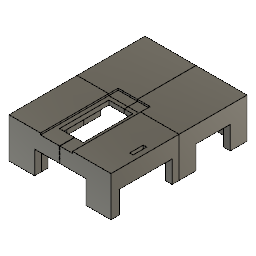
stands for wormbot (v15~recovered) (Autodesk Fusion 360 design; units mm, degrees)
Autodesk Fusion 360 part; units mm, degrees
note: some values were not read from the file. Set by a fixed rule: which face or edge a step refers to.
box "BoxPrimitive1" add length 381 width 305 height 5 placed x (0, 1, 0) y (-1, 0, 0) z (0, 0, 1) at (0, 0, 0) makes body 1
extrude "Extrude1" add 1 faces at (-203.3333, 127, 5) along direction (0, 0, 1) blind 113 on bodies 1 bodies 1
extrude "Extrude2" cut 1 faces at (0, 254, 39.3333) along direction (-1, 0, 0) blind 152.5 on bodies 1 bodies 1
extrude "Extrude3" cut 1 faces at (-203.3333, 0, 39.3333) along direction (0, 1, 0) blind 190.5 on bodies 1 bodies 1
shell "Shell1" thickness 20 removed faces 1 at (-254.1667, 254, 118) on bodies 1
extrude "Extrude4" add 1 faces at (-247.5, 260.6667, 20) along direction (0, 0, 1) blind 20 on bodies 1 bodies 1
sketch "Sketch2" plane through (0, 0, 0) normal (0, 0, 1) x (1, 0, 0)
  line L0 (0, 0) -> (150, 0)
  line L1 (150, 0) -> (150, 200)
  line L2 (150, 200) -> (0, 200)
  line L3 (0, 200) -> (0, 0)
  dimension "d15" = 150
  dimension "d16" = 200
  constraint horizontal L0
  constraint vertical L1
  constraint horizontal L2
  constraint vertical L3
  constraint coincident L0.start L3.end
  measures "d15" distance of L0.start L0.end
  measures "d16" distance of L0 L2
move_body "Move1" bodies 1 to x (1, 0, 0) y (0, 1, 0) z (0, 0, 1) at (110, -190, 0)
extrude "Extrude5" add sketch "Sketch2" along normal blind 118 separate body makes body 2
shell "Shell2" thickness 20 removed faces 1 at (50, 133.3333, 118) on bodies 2
copy_body "CopyPasteBodies1" bodies 2 makes body 3
move_body "Move2" bodies 3 to x (1, 0, 0) y (0, 1, 0) z (0, 0, 1) at (175, 0, 0)
copy_body "CopyPasteBodies2" bodies 3 2 makes body 4 makes body 5
move_body "Move3" bodies 4 5 to x (1, 0, 0) y (0, 1, 0) z (0, 0, 1) at (0, 225, 0)
sketch "Sketch4" plane through (0, 0, 118) normal (0, 0, 1) x (-1, 0, 0)
  line L0 (-20, -405) -> (-130, -405)
  line L1 (-130, -405) -> (-130, -245)
  line L2 (-130, -245) -> (-20, -245)
  line L3 (-20, -245) -> (-20, -405)
  line L4 (0, -425) -> (0, -225)
  line L5 (0, -225) -> (-150, -225)
  line L6 (-150, -225) -> (-150, -425)
  line L7 (-150, -425) -> (0, -425)
  line L8 (-150, -225) -> (-20, -225)
  line L9 (-20, -225) -> (-20, -405)
  line L10 (-20, -405) -> (-150, -405)
  line L11 (-150, -405) -> (-150, -225)
  constraint horizontal L8
  constraint vertical L9
  constraint horizontal L10
  constraint vertical L11
  constraint coincident L0.start L3.end
  constraint coincident L5.end L6.start
sketch "Sketch5" plane through (0, 0, 118) normal (0, 0, 1) x (-1, 0, 0)
  line L0 (-195, -405) -> (-305, -405)
  line L1 (-305, -405) -> (-305, -245)
  line L2 (-305, -245) -> (-195, -245)
  line L3 (-195, -245) -> (-195, -405)
  line L4 (-175, -425) -> (-175, -225)
  line L5 (-175, -225) -> (-325, -225)
  line L6 (-325, -225) -> (-325, -425)
  line L7 (-325, -425) -> (-175, -425)
  line L8 (-175, -225) -> (-305, -225)
  line L9 (-305, -225) -> (-305, -405)
  line L10 (-305, -405) -> (-175, -405)
  line L11 (-175, -405) -> (-175, -225)
  constraint horizontal L8
  constraint vertical L9
  constraint horizontal L10
  constraint vertical L11
  constraint coincident L0.end L1.start
  constraint coincident L4.end L5.start
sketch "Sketch6" plane through (0, 0, 118) normal (0, 0, 1) x (-1, 0, 0)
  line L0 (-20, -180) -> (-130, -180)
  line L1 (-130, -180) -> (-130, -20)
  line L2 (-130, -20) -> (-20, -20)
  line L3 (-20, -20) -> (-20, -180)
  line L4 (0, -200) -> (0, 0)
  line L5 (0, 0) -> (-150, 0)
  line L6 (-150, 0) -> (-150, -200)
  line L7 (-150, -200) -> (0, -200)
  line L8 (-150, -200) -> (-20, -200)
  line L9 (-20, -200) -> (-20, -20)
  line L10 (-20, -20) -> (-150, -20)
  line L11 (-150, -20) -> (-150, -200)
  constraint horizontal L8
  constraint vertical L9
  constraint horizontal L10
  constraint vertical L11
  constraint coincident L2.end L3.start
  constraint coincident L6.end L7.start
sketch "Sketch7" plane through (0, 0, 118) normal (0, 0, 1) x (-1, 0, 0)
  line L0 (-195, -180) -> (-305, -180)
  line L1 (-305, -180) -> (-305, -20)
  line L2 (-305, -20) -> (-195, -20)
  line L3 (-195, -20) -> (-195, -180)
  line L4 (-175, -200) -> (-175, 0)
  line L5 (-175, 0) -> (-325, 0)
  line L6 (-325, 0) -> (-325, -200)
  line L7 (-325, -200) -> (-175, -200)
  line L8 (-175, -200) -> (-305, -200)
  line L9 (-305, -200) -> (-305, -20)
  line L10 (-305, -20) -> (-175, -20)
  line L11 (-175, -20) -> (-175, -200)
  constraint horizontal L8
  constraint vertical L9
  constraint horizontal L10
  constraint vertical L11
  constraint coincident L1.end L2.start
  constraint coincident L4.start L7.end
extrude "Extrude6" cut sketch "Sketch5" sketch "Sketch6" sketch "Sketch4" sketch "Sketch7" against normal blind 100 contours L2 L3 L4 L5 L8 L9 L10 L11 of sketch 2 contours L0 L1 L6 L7 L8 L9 L10 L11 of sketch 3 contours L1 L2 L5 L6 L8 L9 L10 L11 of sketch 4 contours L0 L3 L4 L7 L8 L9 L10 L11 bodies 2 3 4 5
move_body "Move4" bodies 3 2 to x (1, 0, 0) y (0, 1, 0) z (0, 0, 1) at (0, 25, 0)
move_body "Move5" bodies 4 3 to x (1, 0, 0) y (0, 1, 0) z (0, 0, 1) at (-25, 0, 0)
move_body "Move6" bodies 2 4 5 3 to x (1, 0, 0) y (0, -1, 0) z (0, 0, -1) at (-150, 225, 36)
other "Base Mesh Feature1"
move_body "Move7" bodies 5 2 4 3 to x (1, 0, 0) y (0, 1, 0) z (0, 0, 1) at (0, 1.0624, 83.0011)
other "Modify1"
ref_plane "WorkPlane1" through (0, 225, 0) normal (0, 1, 0) x (0, 0, 1)
ref_plane "WorkPlane2" through (0, -600, 0) normal (0, 1, 0) x (0, 0, 1)
ref_plane "WorkPlane3" through (-325, 0, 0) normal (1, 0, 0) x (0, 1, 0)
ref_plane "WorkPlane4" through (0, 0, 650) normal (0, 0, 1) x (1, 0, 0)
ref_plane "WorkPlane5" through (0, 0, -100) normal (0, 0, 1) x (1, 0, 0)
move_body "Move8" bodies 4 3 to x (1, 0, 0) y (0, 1, 0) z (0, 0, 1) at (50, 0, 0)
move_body "Move9" bodies 2 3 to x (1, 0, 0) y (0, 1, 0) z (0, 0, 1) at (0, 70, 0)
extrude "Extrude9" cut 4 faces at (106.6667, 197.7291, 99.0011) (-93.3333, 197.7291, 99.0011) (-93.3333, -125.6042, 99.0011) (106.6667, -125.6042, 99.0011) along direction (0, 0, 1) blind 2 on bodies 2 3 4 5 bodies 2 3 4 5
sketch "Sketch9" plane through (0, -178.9376, 0) normal (0, 1, 0) x (-1, 0, 0)
  line L0 (-180, 101.0011) -> (-180, 1.0011)
  line L1 (-180, 1.0011) -> (-50, 1.0011)
  line L2 (-50, 1.0011) -> (-50, 101.0011)
  line L3 (-50, 101.0011) -> (-180, 101.0011)
  line L4 (-180, 60) -> (-124.686, 101.0011)
  line L5 (-180, 101.0011) -> (-124.686, 101.0011)
  line L6 (-180, 101.0011) -> (-180, 60)
  constraint coincident L0 L4.start
  constraint coincident L3 L4.end
  constraint coincident L0.start L3.end
move_body "Move10" bodies 2 3 to x (1, 0, 0) y (0, 1, 0) z (0, 0, 1) at (0, -70, 0)
move_body "Move11" bodies 3 4 to x (1, 0, 0) y (0, 1, 0) z (0, 0, 1) at (-50, 0, 0)
other "Base Mesh Feature2"
other "Modify2"
sketch "Sketch10" plane through (0, 0, 119.0011) normal (0, 0, 1) x (-1, 0, 0)
  line L0 (150, -1.0624) -> (150, 198.9376)
  line L1 (150, 198.9376) -> (0, 198.9376)
  line L2 (0, 198.9376) -> (0, -1.0624)
  line L3 (0, -1.0624) -> (150, -1.0624)
  line L4 (56.575, -28.8666) -> (-35, -28.8666)
  line L5 (-35, -28.8666) -> (-35, 205)
  line L6 (-35, 205) -> (56.575, 205)
  line L7 (56.575, 205) -> (56.575, -28.8666)
  line L8 (45, 10) -> (-25, 10)
  line L9 (-25, 10) -> (-25, 155)
  line L10 (-25, 155) -> (45, 155)
  line L11 (45, 155) -> (45, 10)
  constraint horizontal L4
  constraint vertical L5
  constraint horizontal L6
  constraint vertical L7
  constraint horizontal L8
  constraint vertical L9
  constraint horizontal L10
  constraint vertical L11
extrude "Extrude10" cut sketch "Sketch10" against normal blind 5 contours L1 L2 L3 L4 L5 L6 L7 L8 L9 L10 | L1 L2 L3 L7 L8 L10 L11 bodies 2 3 4 5
extrude "Extrude11" cut 2 faces at (-30, -106.6667, 119.0011) (8.3333, -106.6667, 119.0011) along direction (0, 0, -1) blind 10 on bodies 4 5 bodies 4 5
extrude "Extrude12" cut 1 faces at (-30, -106.6667, 109.0011) along direction (0, 0, -1) blind 30 on bodies 5 bodies 5
extrude "Extrude13" cut 1 faces at (8.3333, -106.6667, 109.0011) along direction (0, 0, -1) blind 100 on bodies 4 bodies 4
extrude "Extrude14" cut 2 faces at (35, 10.3305, 115.6678) (35, -65.6042, 117.3345) along direction (1, 0, 0) blind 2 on bodies 3 4 bodies 3 4
move_body "Move12" bodies 2 3 4 5 to x (1, 0, 0) y (0, 1, 0) z (0, 0, 1) at (0, 50, 0)
other "Modify3"
sketch "Sketch12" plane through (150, 0, 0) normal (1, 0, 0) x (0, 1, 0)
  line L0 (51.0624, 119.0011) -> (-148.9376, 119.0011)
  line L1 (-148.9376, 119.0011) -> (-148.9376, 1.0011)
  line L2 (-148.9376, 1.0011) -> (51.0624, 1.0011)
  line L3 (51.0624, 1.0011) -> (51.0624, 119.0011)
  line L4 (-129.1971, 16.38) -> (50.8029, 16.38)
  line L5 (50.8029, 16.38) -> (50.8029, 1.38)
  line L6 (50.8029, 1.38) -> (-129.1971, 1.38)
  line L7 (-129.1971, 1.38) -> (-129.1971, 16.38)
  dimension "d65" = 180
  dimension "d66" = 15
  constraint horizontal L4
  constraint vertical L5
  constraint horizontal L6
  constraint vertical L7
  measures "d65" distance of L4.start L4.end
  measures "d66" distance of L4.start L6.end
extrude "Extrude18" cut sketch "Sketch12" against normal blind 30 contours L4 L5 L6 L7 bodies 4
extrude "Extrude19" cut 1 faces at (143.3333, -69.1106, 1.38) along direction (0, 0, -1) blind 10 on bodies 4 bodies 4
sketch "Sketch13" plane through (130, 0, 0) normal (-1, 0, 0) x (0, -1, 0)
  line L0 (-50.8029, 1.0011) -> (-50.8029, 16.38)
  line L1 (-50.8029, 16.38) -> (128.9376, 16.38)
  line L2 (128.9376, 16.38) -> (128.9376, 101.0011)
  line L3 (128.9376, 101.0011) -> (-51.0624, 101.0011)
  line L4 (-51.0624, 101.0011) -> (-51.0624, 1.0011)
  line L5 (-51.0624, 1.0011) -> (-50.8029, 1.0011)
  line L6 (-50.6729, 64.0011) -> (128.9376, 64.0011)
  line L7 (128.9376, 64.0011) -> (128.9376, 59.0011)
  line L8 (128.9376, 59.0011) -> (-50.6729, 59.0011)
  line L9 (-50.6729, 59.0011) -> (-50.6729, 64.0011)
  point P0 (-50.6729, 64.0011)
  dimension "d71" = 5
  constraint horizontal L6
  constraint vertical L7
  constraint horizontal L8
  constraint vertical L9
  constraint coincident P0 L6.start
  measures "d71" distance of P0 L8.end
extrude "Extrude22" cut 1 faces at (143.3333, -69.1106, 16.38) along direction (0, 0, 1) blind 50 on bodies 4 bodies 4
sketch "Pegs 1" plane through (0, 51.0624, 0) normal (0, 1, 0) x (-1, 0, 0)
  line L0 (-37, 114.0011) -> (-37, 119.0011)
  line L1 (-37, 119.0011) -> (-150, 119.0011)
  line L2 (-150, 119.0011) -> (-150, 1.0011)
  line L3 (-150, 1.0011) -> (-130, 1.0011)
  line L4 (-130, 1.0011) -> (-130, 101.0011)
  line L5 (-130, 101.0011) -> (0, 101.0011)
  line L6 (0, 101.0011) -> (0, 114.0011)
  line L7 (0, 114.0011) -> (-37, 114.0011)
  circle A0 centre (-110, 110) radius 5
  circle A1 centre (-140, 79.0011) radius 5
  circle A2 centre (-140, 39.0011) radius 5
  line L8 (0, 20) -> (0, 2.5)
  circle A3 centre (110, 110) radius 5
  circle A4 centre (140, 79.0011) radius 5
  circle A5 centre (140, 39.0011) radius 5
  circle A6 centre (110, 110) radius 4.75
  circle A7 centre (140, 79.0011) radius 4.75
  circle A8 centre (-140, 39.0011) radius 4.75
  circle A9 centre (-110, 110) radius 4.75
  circle A10 centre (-140, 79.0011) radius 4.75
  circle A11 centre (140, 39.0011) radius 4.75
  dimension "d78" = 40
  dimension "d79" = 10
  dimension "d80" = 40
  dimension "d81" = 10
  dimension "d82" = 40
  dimension "d111" = 9.5
  dimension "d112" = 9.5
  dimension "d113" = 9.5
  dimension "d114" = 9.5
  dimension "d115" = 9.5
  dimension "d116" = 9.5
  constraint symmetric A0 L8 A3
  constraint symmetric A1 L8 A4
  constraint symmetric A2 L8 A5
  constraint concentric A3 A6
  constraint concentric A4 A7
  constraint concentric A2 A8
  constraint concentric A0 A9
  constraint concentric A1 A10
  constraint concentric A5 A11
  measures "d78" distance of L2 A0.centre
  measures "d79" diameter of A1
  measures "d80" distance of L1 A1.centre
  measures "d81" diameter of A2
  measures "d82" distance of A1.centre A2.centre
  measures "d111" diameter of A6
  measures "d112" diameter of A7
  measures "d113" diameter of A8
  measures "d114" diameter of A9
  measures "d115" diameter of A10
  measures "d116" diameter of A11
extrude "Extrude23" cut sketch "Pegs 1" along normal blind 10 contours A0 | A1 | A2 | A3 | A4 | A5 | A6 | A7 | A8 | A9 | A10 | A11 bodies 2 3
move_body "Move13" bodies 2 3 to x (1, 0, 0) y (0, 1, 0) z (0, 0, 1) at (0, 50, 0)
extrude "Extrude24" add sketch "Pegs 1" along normal blind 9 contours A6 | A7 | A8 | A9 | A10 | A11 bodies 4 5
move_body "Move14" bodies 2 3 to x (1, 0, 0) y (0, 1, 0) z (0, 0, 1) at (0, -50, 0)
move_body "Move15" bodies 4 3 to x (1, 0, 0) y (0, 1, 0) z (0, 0, 1) at (50, -50.6352, 0.073)
move_body "Move16" bodies 4 5 to x (1, 0, 0) y (0, 1, 0) z (0, 0, 1) at (0, -50, 0)
move_body "Move17" bodies 4 to x (1, 0, 0) y (0, 1, 0) z (0, 0, 1) at (0, 50, 0)
move_body "Move18" bodies 2 to x (1, 0, 0) y (0, 1, 0) z (0, 0, 1) at (0, -50, 0)
sketch "Sketch17" plane through (50, 0, 0) normal (-1, 0, 0) x (0, -1, 0)
  line L0 (-0.4273, 114.0741) -> (-28.2314, 114.0741)
  line L1 (-28.2314, 114.0741) -> (-28.2314, 119.0741)
  line L2 (-28.2314, 119.0741) -> (-200.4273, 119.0741)
  line L3 (-200.4273, 119.0741) -> (-200.4273, 1.0741)
  line L4 (-200.4273, 1.0741) -> (-180.4273, 1.0741)
  line L5 (-180.4273, 1.0741) -> (-180.4273, 101.0741)
  line L6 (-180.4273, 101.0741) -> (-0.4273, 101.0741)
  line L7 (-0.4273, 101.0741) -> (-0.4273, 114.0741)
  circle A0 centre (169.5727, 107.9826) radius 5
  line L8 (199.5727, 114.0741) -> (199.5727, 1.0741)
  circle A1 centre (190, 74.0741) radius 5
  line L9 (199.5727, 114.0741) -> (155.6352, 114.0741)
  circle A2 centre (190.1387, 34.0741) radius 5
  line L10 (0, 2.5) -> (0, 20)
  circle A3 centre (-190.1387, 34.0741) radius 5
  circle A4 centre (-190, 74.0741) radius 5
  circle A5 centre (-169.5727, 107.9826) radius 5
  circle A6 centre (169.5727, 107.9826) radius 3.5
  circle A7 centre (190, 74.0741) radius 3.5
  circle A8 centre (190.1387, 34.0741) radius 3.5
  circle A9 centre (-169.5727, 107.9826) radius 3.5
  circle A10 centre (-190, 74.0741) radius 3.5
  circle A11 centre (-190.1387, 34.0741) radius 3.5
  dimension "d93" = 10
  dimension "d94" = 30
  dimension "d95" = 10
  dimension "d96" = 40
  dimension "d97" = 10
  dimension "d98" = 40
  dimension "d117" = 7
  dimension "d118" = 7
  dimension "d119" = 7
  dimension "d120" = 7
  dimension "d121" = 7
  dimension "d122" = 7
  constraint symmetric A0 L10 A5
  constraint symmetric A1 L10 A4
  constraint symmetric A2 L10 A3
  constraint concentric A0 A6
  constraint concentric A1 A7
  constraint concentric A2 A8
  constraint concentric A5 A9
  constraint concentric A4 A10
  constraint concentric A3 A11
  measures "d93" diameter of A0
  measures "d94" distance of A0.centre L8
  measures "d95" diameter of A1
  measures "d96" distance of A1.centre L9
  measures "d97" diameter of A2
  measures "d98" vertical distance of A1.centre A2.centre
  measures "d117" diameter of A6
  measures "d118" diameter of A7
  measures "d119" diameter of A8
  measures "d120" diameter of A9
  measures "d121" diameter of A10
  measures "d122" diameter of A11
move_body "Move19" bodies 2 5 to x (1, 0, 0) y (0, 1, 0) z (0, 0, 1) at (50, 0, 0)
move_body "Move20" bodies 4 3 to x (1, 0, 0) y (0, 1, 0) z (0, 0, 1) at (0, 0.639, 0)
extrude "Extrude25" cut sketch "Sketch17" along normal blind 10 contours A0 | A1 | A2 | A3 | A4 | A5 | A6 | A7 | A8 | A9 | A10 | A11 bodies 2 5
extrude "Extrude26" add sketch "Sketch17" along normal blind 10 contours A6 | A7 | A8 | A9 | A10 | A11 bodies 3 4
move_body "Move21" bodies 2 4 5 3 to x (1, 0, 0) y (0, -1, 0) z (0, 0, -1) at (0, 2.1325, 128.1482)
move_body "Move22" bodies 3 2 to x (1, 0, 0) y (0, 1, 0) z (0, 0, 1) at (0, -25, 0)
move_body "Move23" bodies 3 4 to x (1, 0, 0) y (0, 1, 0) z (0, 0, 1) at (25, 0, 0)
extrude "Extrude27" add 1 faces at (218.3333, 1.3258, 83.4882) along direction (0, 1, 0) blind 30 on bodies 4 bodies 4
move_body "Move24" bodies 5 3 2 4 to x (1, 0, 0) y (0, -1, 0) z (0, 0, -1) at (0, 2.1402, 124.2941)
move_body "Move25" bodies 2 3 4 5 to x (1, 0, 0) y (0, 1, 0) z (0, 0, 1) at (-49.8589, 23.9323, 0)
move_body "Move26" bodies 2 3 to x (1, 0, 0) y (0, 1, 0) z (0, 0, 1) at (0, -25, 0)
move_body "Move27" bodies 4 3 to x (1, 0, 0) y (0, 1, 0) z (0, 0, 1) at (-25, 0, 0)
move_body "Move28" bodies 2 5 3 4 to x (1, 0, 0) y (0, 1, 0) z (0, 0, 1) at (-1.1259, 26.5865, 0)
sketch "Sketch18" plane through (0, 0, 0) normal (0, 0, 1) x (1, 0, 0)
  line L0 (-266.1691, -475) -> (159.4864, -475)
  line L1 (159.4864, -475) -> (159.4864, 284.4296)
  line L2 (159.4864, 284.4296) -> (-266.1691, 284.4296)
  line L3 (-266.1691, 284.4296) -> (-266.1691, -475)
  constraint horizontal L0
  constraint vertical L1
  constraint horizontal L2
  constraint vertical L3
other "Base Mesh Feature4"
other "Modify4"
other "Base Mesh Feature5"
other "Modify5"
extrude "Extrude28" add sketch "Sketch18" against normal blind 30 separate body makes body 6
extrude "Extrude29" add 1 faces at (159.4864, -221.8568, -10) along direction (1, 0, 0) blind 50 on bodies 6 bodies 6
sketch "Sketch19" plane through (0, 0, 0) normal (0, 0, 1) x (1, 0, 0)
  line L0 (-258.0781, -43.3) -> (-233.0723, -43.3)
  line L1 (-233.0723, -43.3) -> (-233.0723, -17.8396)
  line L2 (-233.0723, -17.8396) -> (-258.0781, -17.8396)
  line L3 (-258.0781, -17.8396) -> (-258.0781, -43.3)
  constraint horizontal L0
  constraint vertical L1
  constraint horizontal L2
  constraint vertical L3
extrude "Extrude30" add sketch "Sketch19" along normal blind 15 separate body makes body 7
move_body "Move29" bodies 3 4 to x (1, 0, 0) y (0, 1, 0) z (0, 0, 1) at (30, 0, 0)
move_body "Move30" bodies 2 3 to x (1, 0, 0) y (0, 1, 0) z (0, 0, 1) at (0, 40, 0)
move_body "Move31" bodies 2 3 4 5 to x (1, 0, 0) y (0, -1, 0) z (0, 0, -1) at (0, 183.1777, -5.7059)
move_body "Move32" bodies 4 5 to x (1, 0, 0) y (0, 1, 0) z (0, 0, 1) at (0, -40, 0)
move_body "Move33" bodies 4 3 to x (1, 0, 0) y (0, 1, 0) z (0, 0, 1) at (-30, 0, 0)
move_body "Move34" bodies 2 4 5 3 to x (1, 0, 0) y (0, -1, 0) z (0, 0, -1) at (0, 143.1777, -5.7059)
sketch "Sketch20" plane through (0, -148.4112, 0) normal (0, -1, 0) x (1, 0, 0)
  line L0 (-0.9847, 110.1471) -> (-57.5597, 110.1471)
  line L1 (-57.5597, 110.1471) -> (-57.5597, 115.1471)
  line L2 (-57.5597, 115.1471) -> (-150.9847, 115.1471)
  line L3 (-150.9847, 115.1471) -> (-150.9847, -2.8529)
  line L4 (-150.9847, -2.8529) -> (-0.9847, -2.8529)
  line L5 (-0.9847, -2.8529) -> (-0.9847, 110.1471)
  line L6 (0, 0) -> (-75, 0)
  line L7 (-75, 0) -> (-75, 65.379)
  line L8 (-75, 65.379) -> (0, 65.379)
  line L9 (0, 65.379) -> (0, 0)
  line L10 (0, 0) -> (75, 0)
  line L11 (75, 0) -> (75, 65.379)
  line L12 (75, 65.379) -> (0, 65.379)
  line L13 (0, 65.379) -> (0, 0)
  dimension "d123" = 75
  dimension "d124" = 75
  dimension "d125" = 65.379
  dimension "d126" = 65.379
  constraint horizontal L6
  constraint vertical L7
  constraint horizontal L8
  constraint vertical L9
  constraint coincident L6.start L9.end
  constraint horizontal L10
  constraint vertical L11
  constraint horizontal L12
  constraint vertical L13
  measures "d123" distance of L6.start L6.end
  measures "d124" distance of L6.start L10.end
  measures "d125" distance of L6 L8
  measures "d126" distance of L10 L12
extrude "Extrude31" cut sketch "Sketch20" against normal blind 90 contours L5 L6 L7 L8 | L9 L10 L11 L12 L13 bodies 4 5
extrude "Extrude32" cut 1 faces at (0, -135.074, 43.586) along direction (-1, 0, 0) blind 5 on bodies 4 bodies 4
extrude "Extrude33" cut 2 faces at (-25.6565, -141.7445, 0) (49.6718, -135.074, 0) along direction (0, 0, -1) blind 10 on bodies 4 5 bodies 4 5
sketch "Sketch21" plane through (0, 0, 0) normal (0, 0, 1) x (1, 0, 0)
  circle A0 centre (-7.8893, -314.0254) radius 164
  circle A1 centre (-7.8893, -314.0254) radius 86
  dimension "d133" = 328
  dimension "d134" = 172
  constraint concentric A0 A1
  measures "d133" diameter of A0
  measures "d134" diameter of A1
extrude "Extrude34" add sketch "Sketch21" along normal blind 120 separate body makes body 8
other "Base Mesh Feature6"
move_body "Move35" bodies 3 4 to x (1, 0, 0) y (0, 1, 0) z (0, 0, 1) at (20, 0, 0)
extrude "Extrude35" cut 2 faces at (9.0153, -140.201, 71.4799) (9.0153, -120.1611, 103.7847) along direction (1, 0, 0) blind 10 on bodies 4 bodies 4
extrude "Extrude36" add 2 faces at (-10.9847, -140.7442, 72.1456) (-10.9847, -120.6389, 104.6198) along direction (1, 0, 0) blind 10 on bodies 5 bodies 5
move_body "Move36" bodies 4 3 to x (1, 0, 0) y (0, 1, 0) z (0, 0, 1) at (-20, 0, 0)
sketch "Sketch22" plane through (0, -148.4112, 0) normal (0, -1, 0) x (1, 0, 0)
  line L0 (-75, -2.8529) -> (-75, 65.379)
  line L1 (-75, 65.379) -> (-0.9847, 65.379)
  line L2 (-0.9847, 65.379) -> (-0.9847, 110.1471)
  line L3 (-0.9847, 110.1471) -> (-57.5597, 110.1471)
  line L4 (-57.5597, 110.1471) -> (-57.5597, 115.1471)
  line L5 (-57.5597, 115.1471) -> (-150.9847, 115.1471)
  line L6 (-150.9847, 115.1471) -> (-150.9847, -2.8529)
  line L7 (-150.9847, -2.8529) -> (-75, -2.8529)
  line L8 (-3, 109) -> (-3, 99)
  line L9 (-3, 99) -> (-1, 102.4641)
  line L10 (-3, 109) -> (-1, 105.5359)
  line L11 (-1, 105.5359) -> (-1, 102.4641)
  line L12 (-2.9901, 95.9334) -> (-0.9992, 92.4641)
  line L13 (-2.9901, 95.9334) -> (-2.9915, 85.9334)
  line L14 (-2.9915, 85.9334) -> (-0.9995, 89.4021)
  line L15 (-0.9992, 92.4641) -> (-0.9995, 89.4021)
  line L16 (-2.9682, 82.8833) -> (-0.998, 79.4021)
  line L17 (-2.9682, 82.8833) -> (-2.9835, 72.8833)
  line L18 (-2.9835, 72.8833) -> (-0.9954, 76.3542)
  line L19 (-0.998, 79.4021) -> (-0.9954, 76.3542)
  dimension "d143" = 10
  dimension "d145" = 4
  dimension "d146" = 4
  dimension "d148" = 10
  dimension "d149" = 4
  dimension "d150" = 4
  dimension "d151" = 10
  dimension "d152" = 10
  dimension "d153" = 4
  dimension "d154" = 4
  dimension "d155" = 10
  measures "d143" distance of L8.start L8.end
  measures "d145" distance of L8.end L9.end
  measures "d146" distance of L8.start L10.end
  measures "d148" distance of L13.end L12.start
  measures "d149" distance of L14.end L13.end
  measures "d150" distance of L12.end L12.start
  measures "d151" distance of L9.end L12.end
  measures "d152" distance of L17.end L16.start
  measures "d153" distance of L18.end L17.end
  measures "d154" distance of L16.end L16.start
  measures "d155" vertical distance of L14.end L16.end
extrude "Extrude37" cut sketch "Sketch22" against normal blind 55 contours L8 L9 L10 L11 | L12 L13 L14 L15 | L16 L17 L18 L19 bodies 5
extrude "Extrude38" cut 1 faces at (-0.9971, -141.7445, 78.3862) along direction (1, 0, 0.000852) blind 21 on bodies 5 bodies 5
extrude "Extrude39" cut 1 faces at (-0.9993, -141.7445, 91.4434) along direction (1, 0, -0.000089) blind 6 on bodies 5 bodies 5
extrude "Extrude40" cut 1 faces at (-1, -119.1194, 104.512) along direction (1, 0, 0) blind 16 on bodies 5 bodies 5
extrude "Extrude41" add sketch "Sketch22" against normal blind 20 separate body contours L8 L9 L10 L11 | L12 L13 L14 L15 | L16 L17 L18 L19 makes body 9 at (-2.9733, -141.7445, 79.5499) makes body 10 at (-2.9906, -141.7445, 92.6001) makes body 11 at (-3, -141.7445, 105.6667)
extrude "Extrude42" add 1 faces at (-2.3333, -128.4112, 103.488) along direction (0, 1, 0) blind 24 on bodies 11 bodies 11
sketch "Sketch23" plane through (0, 251.5888, 0) normal (0, 1, 0) x (-1, 0, 0)
  line L0 (150.9847, 115.1471) -> (0.9847, 115.1471)
  line L1 (0.9847, 115.1471) -> (0.9847, -2.8529)
  line L2 (0.9847, -2.8529) -> (150.9847, -2.8529)
  line L3 (150.9847, -2.8529) -> (150.9847, 115.1471)
  line L4 (-1.0155, 113.9873) -> (0.9845, 110.5232)
  line L5 (-1.0155, 113.9873) -> (-1.0155, 103.9873)
  line L6 (0.9845, 110.5232) -> (0.9845, 107.4514)
  line L7 (-1.0155, 103.9873) -> (0.9845, 107.4514)
  line L8 (-1.0055, 100.9208) -> (0.9853, 97.4514)
  line L9 (-1.0055, 100.9208) -> (-1.007, 90.9208)
  line L10 (0.9853, 97.4514) -> (0.9851, 94.3895)
  line L11 (-1.007, 90.9208) -> (0.9851, 94.3895)
  line L12 (-0.9837, 87.8706) -> (0.9865, 84.3895)
  line L13 (-0.9837, 87.8706) -> (-0.999, 77.8706)
  line L14 (-0.999, 77.8706) -> (0.9891, 81.3415)
  line L15 (0.9865, 84.3895) -> (0.9891, 81.3415)
  line L16 (-1, 39) -> (1, 35.5359)
  line L17 (-1, 39) -> (-1, 29)
  line L18 (1, 35.5359) -> (1, 32.4641)
  line L19 (-1, 29) -> (1, 32.4641)
  line L20 (-0.9901, 25.9334) -> (1.0008, 22.4641)
  line L21 (-0.9901, 25.9334) -> (-0.9915, 15.9334)
  line L22 (1.0008, 22.4641) -> (1.0005, 19.4021)
  line L23 (-0.9915, 15.9334) -> (1.0005, 19.4021)
  line L24 (-0.9682, 12.8833) -> (1.002, 9.4021)
  line L25 (-0.9682, 12.8833) -> (-0.9835, 2.8833)
  line L26 (-0.9835, 2.8833) -> (1.0046, 6.3542)
  line L27 (1.002, 9.4021) -> (1.0046, 6.3542)
  dimension "d170" = 10
  dimension "d171" = 4
  dimension "d172" = 4
  dimension "d173" = 10
  dimension "d174" = 4
  dimension "d175" = 4
  dimension "d176" = 10
  dimension "d177" = 10
  dimension "d178" = 4
  dimension "d179" = 4
  dimension "d180" = 10
  dimension "d181" = 10
  dimension "d182" = 4
  dimension "d183" = 4
  dimension "d184" = 10
  dimension "d185" = 4
  dimension "d186" = 4
  dimension "d187" = 10
  dimension "d188" = 10
  dimension "d189" = 4
  dimension "d190" = 4
  dimension "d191" = 10
  measures "d170" distance of L4.start L5.end
  measures "d171" distance of L5.end L6.end
  measures "d172" distance of L4.start L4.end
  measures "d173" distance of L9.end L8.start
  measures "d174" distance of L10.end L9.end
  measures "d175" distance of L8.end L8.start
  measures "d176" distance of L6.end L8.end
  measures "d177" distance of L12.start L13.end
  measures "d178" distance of L13.end L14.end
  measures "d179" distance of L12.start L12.end
  measures "d180" vertical distance of L10.end L12.end
  measures "d181" distance of L16.start L17.end
  measures "d182" distance of L17.end L18.end
  measures "d183" distance of L16.start L16.end
  measures "d184" distance of L21.end L20.start
  measures "d185" distance of L22.end L21.end
  measures "d186" distance of L20.end L20.start
  measures "d187" distance of L18.end L20.end
  measures "d188" distance of L24.start L25.end
  measures "d189" distance of L25.end L26.end
  measures "d190" distance of L24.start L24.end
  measures "d191" vertical distance of L22.end L24.end
move_body "Move41" bodies 2 to x (1, 0, 0) y (0, 1, 0) z (0, 0, 1) at (-30, 0, 0)
extrude "Extrude43" cut 3 faces at (-10.9847, 239.9377, 31.4799) (-10.9847, 239.799, 71.4799) (-10.9847, 219.3717, 105.3885) along direction (1, 0, 0) blind 10 on bodies 3 bodies 3
extrude "Extrude44" add 3 faces at (-40.9847, 240.0562, 28.1718) (-40.9847, 239.1494, 70.6621) (-40.9847, 218.7221, 104.5706) along direction (1, 0, 0) blind 10 on bodies 2 bodies 2
extrude "Extrude45" cut sketch "Sketch23" against normal blind 200 contours L1 L24 L25 L26 | L1 L8 L9 L10 L11 | L1 L20 L21 L23 | L1 L12 L13 L14 | L1 L16 L17 L19 bodies 3
extrude "Extrude46" cut 3 faces at (0.3384, 251.5888, 33.4792) (0.3323, 251.5888, 21.453) (0.3326, 251.5888, 83.3769) along direction (0, 1, 0) blind 3 on bodies 3 bodies 3
extrude "Extrude47" cut 1 faces at (0.3223, 251.5888, 8.3997) along direction (0, 1, 0) blind 4 on bodies 3 bodies 3
extrude "Extrude48" cut 1 faces at (0.3426, 251.5888, 96.431) along direction (0, 1, 0) blind 11 on bodies 3 bodies 3
move_body "Move42" bodies 2 to x (1, 0, 0) y (0, 1, 0) z (0, 0, 1) at (30, 0, 0)
extrude "Extrude49" add sketch "Sketch23" against normal blind 20 contours L1 L24 L25 L26 | L1 L8 L9 L10 L11 | L1 L20 L21 L23 | L1 L12 L13 L14 | L1 L16 L17 L19 bodies 2
move_body "Move43" bodies 3 2 to x (1, 0, 0) y (0, 1, 0) z (0, 0, 1) at (0, 120, 0)
sketch "Sketch24" plane through (0, -128.4073, 0) normal (0, 1, 0) x (-1, 0, 0)
  line L0 (-75, -2.78) -> (-75, 65.379)
  line L1 (-75, 65.379) -> (0.9847, 65.379)
  line L2 (0.9847, 65.379) -> (0.9847, 97.22)
  line L3 (0.9847, 97.22) -> (-129.0153, 97.22)
  line L4 (-129.0153, 97.22) -> (-129.0153, 62.5989)
  line L5 (-129.0153, 62.5989) -> (-119.0153, 62.5989)
  line L6 (-119.0153, 62.5989) -> (-119.0153, -2.78)
  line L7 (-119.0153, -2.78) -> (-75, -2.78)
  line L8 (-75, -2.78) -> (-85, -2.78)
  line L9 (-85, -2.78) -> (-85, 97.22)
  line L10 (-85, 97.22) -> (-75, 97.22)
  line L11 (-75, 97.22) -> (-75, -2.78)
  line L12 (75, -2.8529) -> (85, -2.8529)
  line L13 (85, -2.8529) -> (85, 97.1471)
  line L14 (85, 97.1471) -> (75, 97.1471)
  line L15 (75, 97.1471) -> (75, -2.8529)
  point P0 (75, -2.8529)
  dimension "d206" = 10
  dimension "d207" = 10
  constraint horizontal L8
  constraint vertical L9
  constraint horizontal L10
  constraint vertical L11
  constraint coincident L0.start L7.end
  constraint horizontal L12
  constraint vertical L13
  constraint horizontal L14
  constraint vertical L15
  constraint coincident P0 L12.start
  measures "d206" distance of L0.start L8.end
  measures "d207" distance of P0 L12.end
extrude "Extrude50" add sketch "Sketch24" along normal blind 20 contours L0 L3 L7 L8 L9 L10 L11 | L12 L13 L14 L15 bodies 4 5 9 10 11
extrude "Extrude51" cut 1 faces at (142.3486, 21.3332, 40.806) along direction (0, 1, 0) blind 10 on bodies 4 bodies 4
extrude "Extrude52" cut 1 faces at (96.3384, -128.4073, 52.3463) along direction (0, -1, 0) blind 10 on bodies 4 bodies 4
extrude "Extrude53" cut 1 faces at (132.3486, -128.6668, 19.013) along direction (0, -1, 0) blind 10 on bodies 4 bodies 4
sketch "Sketch25" plane through (0, 0, 115.22) normal (0, 0, 1) x (-1, 0, 0)
  line L0 (-36.0153, -51.5927) -> (-36.0153, 148.4073)
  line L1 (-36.0153, 148.4073) -> (-149.0153, 148.4073)
  line L2 (-149.0153, 148.4073) -> (-149.0153, -51.5927)
  line L3 (-149.0153, -51.5927) -> (-36.0153, -51.5927)
  line L4 (-124.0153, 28.4073) -> (-134.0153, 28.4073)
  line L5 (-134.0153, 28.4073) -> (-134.0153, 68.4073)
  line L6 (-134.0153, 68.4073) -> (-124.0153, 68.4073)
  line L7 (-124.0153, 68.4073) -> (-124.0153, 28.4073)
  dimension "d216" = 10
  dimension "d217" = 40
  dimension "d218" = 15
  dimension "d219" = 80
  constraint horizontal L4
  constraint vertical L5
  constraint horizontal L6
  constraint vertical L7
  measures "d216" distance of L4.start L4.end
  measures "d217" distance of L4.start L6.end
  measures "d218" distance of L2 L5
  measures "d219" distance of L1 L6
extrude "Extrude54" cut sketch "Sketch25" against normal blind 100 contours L4 L5 L6 L7 bodies 4
move_body "Move44" bodies 2 3 to x (1, 0, 0) y (0, 1, 0) z (0, 0, 1) at (0, -120, 0)
sketch "Sketch26" plane through (-150.9847, 0, 0) normal (-1, 0, 0) x (0, -1, 0)
  line L0 (148.4112, 115.1471) -> (-51.5888, 115.1471)
  line L1 (-51.5888, 115.1471) -> (-51.5888, -2.8529)
  line L2 (-51.5888, -2.8529) -> (148.4112, -2.8529)
  line L3 (148.4112, -2.8529) -> (148.4112, 115.1471)
  line L4 (-1.5888, -2.8529) -> (98.4112, -2.8529)
  line L5 (98.4112, -2.8529) -> (98.4112, 65.1471)
  line L6 (98.4112, 65.1471) -> (-1.5888, 65.1471)
  line L7 (-1.5888, 65.1471) -> (-1.5888, -2.8529)
  line L8 (-201.5888, -2.78) -> (-101.5888, -2.78)
  line L9 (-101.5888, -2.78) -> (-101.5888, 65.22)
  line L10 (-101.5888, 65.22) -> (-201.5888, 65.22)
  line L11 (-201.5888, 65.22) -> (-201.5888, -2.78)
  line L12 (-251.5927, -2.78) -> (-51.5927, -2.78)
  dimension "d222" = 100
  dimension "d223" = 68
  dimension "d224" = 50
  dimension "d225" = 100
  dimension "d226" = 68
  dimension "d227" = 50
  constraint horizontal L4
  constraint vertical L5
  constraint horizontal L6
  constraint vertical L7
  constraint coincident L2 L4.start
  constraint horizontal L8
  constraint vertical L9
  constraint horizontal L10
  constraint vertical L11
  constraint coincident L8.start L12
  measures "d222" distance of L4.start L4.end
  measures "d223" distance of L4.start L6.end
  measures "d224" distance of L3 L5
  measures "d225" distance of L8.start L8.end
  measures "d226" distance of L8.start L10.end
  measures "d227" distance of L1 L9
extrude "Extrude55" cut sketch "Sketch26" against normal blind 20 contours L2 L4 L5 L6 L7 | L8 L9 L10 L11 L12 bodies 2 5
extrude "Extrude56" cut 1 faces at (-144.3181, 168.2555, -2.78) along direction (0, 0, -1) blind 20 on bodies 2 bodies 2
extrude "Extrude57" cut sketch "Sketch26" against normal blind 450 contours L8 L9 L10 L11 L12 bodies 3
extrude "Extrude58" add 1 faces at (139.0153, -138.6668, 40.806) along direction (0, 1, 0) blind 15 on bodies 4 bodies 4
extrude "Extrude59" add 1 faces at (96.3384, -138.4073, 52.3463) along direction (0, 1, 0) blind 15 on bodies 4 bodies 4
other "Base Mesh Feature7"
other "Modify6"
sketch "Sketch27" plane through (0, 0, 115.22) normal (0, 0, 1) x (-1, 0, 0)
  line L0 (-36.0153, -79.3969) -> (-36.0153, -51.5927)
  line L1 (-36.0153, -51.5927) -> (-149.0153, -51.5927)
  line L2 (-149.0153, -51.5927) -> (-149.0153, -251.5927)
  line L3 (-149.0153, -251.5927) -> (0.9847, -251.5927)
  line L4 (0.9847, -251.5927) -> (0.9847, -79.3969)
  line L5 (0.9847, -79.3969) -> (-36.0153, -79.3969)
  line L6 (52.2706, -32.0965) -> (41.5539, -32.0965)
  line L7 (41.5539, -32.0965) -> (41.5539, 95.6595)
  line L8 (41.5539, 95.6595) -> (52.2706, 95.6595)
  line L9 (52.2706, 95.6595) -> (52.2706, -32.0965)
  line L10 (-19.8881, 95.6595) -> (-31.2799, 95.6595)
  line L11 (-31.2799, 95.6595) -> (-31.2799, -32.0965)
  line L12 (-31.2799, -32.0965) -> (-19.8881, -32.0965)
  line L13 (-19.8881, -32.0965) -> (-19.8881, 95.6595)
  constraint horizontal L6
  constraint vertical L7
  constraint horizontal L8
  constraint vertical L9
  constraint horizontal L10
  constraint vertical L11
  constraint horizontal L12
  constraint vertical L13
extrude "Extrude60" add sketch "Sketch27" along normal blind 40 separate body contours L6 L7 L8 L9 | L10 L11 L12 L13 makes body 12 at (-41.5539, -53.0742, 141.8867) makes body 13 at (19.8881, -53.0742, 141.8867)
other "Modify7"
hidden bodies 1 6 7 8 12 13
named bodies: "OG Box", "Top Left Box", "Top Right Box", "Bottom Right Box", "Bottom Left Box", "DT3", "DT2", "DT1"
